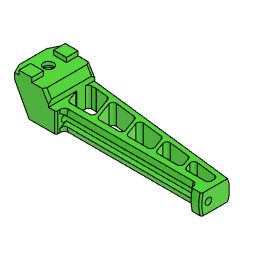
Single Piece Spool Holder v23 (Autodesk Fusion 360 design; units mm, degrees)
Autodesk Fusion 360 part; units mm, degrees
sketch "Sketch1" plane through (0, 0, 0) normal (0, 1, 0) x (1, 0, 0)
  line L0 (0, 0) -> (123.25, 0)
  line L1 (123.25, 0) -> (123.25, -30)
  line L2 (123.25, -30) -> (0, -30)
  line L3 (0, -30) -> (0, 0)
  line L4 (10, -30) -> (10, 0) construction
  line L5 (25, -30) -> (25, 0) construction
  dimension "d2" = 30
  dimension "d39" = 10
  dimension "d40" = 15
  dimension "d74" = 123.25
  constraint horizontal L0
  constraint vertical L1
  constraint horizontal L2
  constraint vertical L3
  constraint coincident L0.start L3.end
  constraint coincident L2 L4.start
  constraint coincident L0 L4.end
  constraint perpendicular L0 L4
  constraint coincident L2 L5.start
  constraint coincident L0 L5.end
  constraint perpendicular L0 L5
  measures "d2" distance of L0.start L2.end
  measures "d39" distance of L3 L4
  measures "d40" distance of L4 L5
  measures "d74" distance of L1 L3
extrude "Extrude1" add sketch "Sketch1" along normal mid plane 13 makes body 1
sketch "Sketch7" plane through (0, 6.5, 0) normal (0, 1, 0) x (-1, 0, 0)
  line L0 (0, 30) -> (-123.25, 30)
  line L1 (-123.25, 30) -> (-123.25, 0)
  line L2 (-123.25, 0) -> (0, 0)
  line L3 (0, 0) -> (0, 30)
  line L4 (0, 30) -> (-25, 30)
  line L5 (-25, 30) -> (-25, 0)
  line L6 (-25, 0) -> (0, 0)
  line L7 (0, 0) -> (0, 30)
  dimension "d75" = 25
  constraint horizontal L4
  constraint vertical L5
  constraint horizontal L6
  constraint vertical L7
  constraint coincident L2 L5.end
  constraint coincident L0.start L3.end
  measures "d75" distance of L0.start L4.end
extrude "Extrude9" add sketch "Sketch7" along normal blind 8.5 contours L0 L2 L3 L4 L5 L6 L7 bodies 1
sketch "Sketch2" plane through (0, 0, 0) normal (0, 0, 1) x (1, 0, 0)
  line L0 (0, -6.5) -> (0, 15)
  line L1 (25, 6.5) -> (123.25, 6.5)
  line L2 (123.25, 6.5) -> (123.25, -6.5)
  line L3 (123.25, -6.5) -> (0, -6.5)
  line L4 (5.825, 15) -> (14.175, 15)
  line L5 (14.175, 15) -> (14.175, 17.8)
  line L6 (14.175, 17.8) -> (5.825, 17.8)
  line L7 (5.825, 17.8) -> (5.825, 15)
  line L8 (10, 17.8) -> (10, 15) construction
  line L9 (0, 15) -> (25, 15)
  line L10 (25, 15) -> (25, 6.5)
  dimension "d20" = 10
  dimension "d21" = 2.8
  dimension "d22" = 8.35
  constraint horizontal L4
  constraint vertical L5
  constraint horizontal L6
  constraint vertical L7
  constraint midpoint L6 L8.start
  constraint midpoint L4 L8.end
  constraint coincident L9 L4.start
  constraint coincident L4.start L7.end
  measures "d20" distance of L0.end L8
  measures "d21" distance of L4.end L5.end
  measures "d22" distance of L5.end L6.end
extrude "Extrude2" add sketch "Sketch2" along normal blind 30 contours L4 L5 L6 L7 L9 bodies 1
sketch "Sketch3" plane through (0, -6.5, 0) normal (0, -1, 0) x (-1, 0, 0)
  line L0 (-10, -30) -> (-10, 0) construction
  circle A0 centre (-10, -15) radius 3.25
  line L1 (-123.25, -30) -> (0, -30)
  line L2 (0, -30) -> (0, 0)
  line L3 (0, 0) -> (-123.25, 0)
  line L4 (-123.25, 0) -> (-123.25, -30)
  line L5 (-14.175, 0) -> (-5.825, 0)
  line L6 (-5.825, 0) -> (-5.825, -30)
  line L7 (-5.825, -30) -> (-14.175, -30)
  line L8 (-14.175, -30) -> (-14.175, 0)
  dimension "d14" = 6.5
  constraint midpoint L0 A0.centre
  constraint midpoint L0.start L7
  constraint midpoint L0.end L5
  measures "d14" diameter of A0
extrude "Extrude3" cut sketch "Sketch3" against normal through all contours A0 bodies 1
sketch "Sketch4" plane through (0, -6.5, 0) normal (0, -1, 0) x (-1, 0, 0)
  circle A0 centre (-10, -15) radius 6.5
  circle A1 centre (-10, -15) radius 3.25
  line L0 (-123.25, -30) -> (0, -30)
  line L1 (0, -30) -> (0, 0)
  line L2 (0, 0) -> (-123.25, 0)
  line L3 (-123.25, 0) -> (-123.25, -30)
  dimension "d16" = 13
  constraint coincident A0.centre A1.centre
  measures "d16" diameter of A0
extrude "Extrude4" cut sketch "Sketch4" against normal up to surface (16 mm away) contours A0 | A1 bodies 1
chamfer "Chamfer1" distance 3.25 angle 45 1 edges at (13.0301, 9.5, 16.1753) on bodies 1
ref_plane "WorkPlane1" through (61.625, 5.65, 15) normal (0, 0, 1) x (1, 0, 0)
sketch "Sketch5" plane through (123.25, 0, 0) normal (1, 0, 0) x (0, 1, 0)
  line L0 (-6.5, 0) -> (6.5, 0)
  line L1 (6.5, 0) -> (6.5, 30)
  line L2 (6.5, 30) -> (-6.5, 30)
  line L3 (-6.5, 30) -> (-6.5, 0)
  circle A0 centre (0, 5.7) radius 20
  circle A1 centre (0, 5.7) radius 24
  line L4 (0, 0) -> (0, 30) construction
  circle A2 centre (0, 24.4) radius 2.1
  line L5 (-6.5, 0) -> (6.5, 0)
  line L6 (6.5, 0) -> (6.5, 30)
  line L7 (6.5, 30) -> (-6.5, 30)
  line L8 (-6.5, 30) -> (-6.5, 0)
  point P0 (27.1204, 5.059)
  point P1 (24.0412, 4.3321)
  point P2 (14.8796, 5.059)
  point P3 (17.9588, 4.3321)
  dimension "d86" = 40
  dimension "d87" = 48
  dimension "d88" = 5.7
  dimension "d89" = 24.4
  dimension "d90" = 4.2
  constraint coincident L4.start origin
  constraint midpoint L2 L4.end
  constraint coincident A0.centre A1.centre
  constraint coincident A0.centre L4
  constraint coincident L4 A2.centre
  measures "d86" diameter of A0
  measures "d87" diameter of A1
  measures "d88" distance of L0 A0.centre
  measures "d89" distance of L4.start A2.centre
  measures "d90" diameter of A2
extrude "Extrude5" cut sketch "Sketch5" against normal blind 86.25 from surface at -7 contours L1 L3 A0 A1 A2 L6 L8 | L1 L2 L3 A1 L6 L7 L8 | A0 A2 picked at (-0.0509, 25.9594) bodies 1
extrude "Extrude6" cut sketch "Sketch5" against normal blind 7 contours L1 L2 L3 A1 L6 L7 L8 bodies 1
extrude "Extrude7" cut sketch "Sketch5" against normal up to surface (100.25 mm away) contours A0 A2 | A0 A2 bodies 1
chamfer "Chamfer2" distance 1.3 distance2 2.2 2 edges at (73.125, -1.7041, 25.6273) (73.125, 1.7041, 25.6273) measured on face at (58.75, -5.4581, 24.9408) measured on face at (58.75, 2.2474, 25.5733) on bodies 1
fillet "Fillet1" radius 1 3 edges at (123.25, 0, 29.7) (116.25, 0, 29.7) (30, 0, 30) on bodies 1
chamfer "Chamfer3" distance 3 distance2 6 2 edges at (0, 4.25, 30) (0, 4.25, 0) measured on face at (18, -2.1667, 30) measured on face at (49.4167, -2.1667, 0) on bodies 1
chamfer "Chamfer4" distance 11 distance2 93 1 edges at (123.25, 0, 0) measured on face at (123.25, 0.0523, 7.4353) on bodies 1
sketch "Sketch6" plane through (0, -6.5, 0) normal (0, -1, 0) x (1, 0, 0)
  line L0 (30, 24.6143) -> (30, 29)
  line L1 (29, 30) -> (3, 30)
  line L2 (3, 30) -> (0, 24)
  line L3 (0, 24) -> (0, 6)
  line L4 (0, 6) -> (3, 0)
  line L5 (3, 0) -> (30.25, 0)
  circle A0 centre (10, 15) radius 6.5
  line L6 (31.5445, 30) -> (20.6254, 0)
  line L7 (29.4161, 30) -> (18.497, 0)
  line L8 (0, 0) -> (128.5239, 0)
  line L9 (128.5239, 0) -> (128.5239, 30)
  line L10 (128.5239, 30) -> (0, 30)
  line L11 (0, 30) -> (0, 0)
  line L12 (48.4161, 30) -> (37.497, 0)
  line L13 (50.5445, 30) -> (39.6254, 0)
  line L14 (67.4161, 30) -> (56.497, 0)
  line L15 (69.5445, 30) -> (58.6254, 0)
  line L16 (86.4161, 30) -> (75.497, 0)
  line L17 (88.5445, 30) -> (77.6254, 0)
  line L18 (105.4161, 30) -> (94.497, 0)
  line L19 (107.5445, 30) -> (96.6254, 0)
  arc A1 (30, 29) -> (29, 30) centre (29, 29) ccw
  line L20 (30.25, 0) -> (123.25, 11)
  line L21 (123.25, 11) -> (123.25, 27.7624)
  spline S0 degree 3 poles (122.25, 28.803) (122.3719, 28.803) (122.5152, 28.7737) (122.7418, 28.6777) (122.8647, 28.5932) (123.0406, 28.4132) (123.1238, 28.285) (123.2204, 28.0461) (123.25, 27.8927) (123.25, 27.7624) knots 0.605058 0.605058 0.605058 0.605058 0.64162 0.64162 0.678904 0.678904 0.71712 0.71712 0.756197 0.756197 0.756197 0.756197
  line L22 (122.25, 28.803) -> (117.25, 28.803)
  spline S1 degree 3 poles (116.25, 27.7624) (116.25, 27.8927) (116.2796, 28.0461) (116.3762, 28.285) (116.4594, 28.4132) (116.6353, 28.5932) (116.7582, 28.6777) (116.9848, 28.7737) (117.1281, 28.803) (117.25, 28.803) knots 0.453919 0.453919 0.453919 0.453919 0.492996 0.492996 0.531212 0.531212 0.568496 0.568496 0.605058 0.605058 0.605058 0.605058
  line L23 (116.25, 27.7624) -> (116.25, 24.6143)
  line L24 (116.25, 24.6143) -> (30, 24.6143)
  line L25 (119.25, 14.5548) -> (119.25, 20.6143)
  line L26 (119.25, 20.6143) -> (26, 20.6143)
  line L27 (26, 20.6143) -> (26, 26)
  line L28 (26, 26) -> (5.4721, 26)
  line L29 (5.4721, 26) -> (4, 23.0557)
  line L30 (4, 23.0557) -> (4, 6.9443)
  line L31 (4, 6.9443) -> (5.4721, 4)
  line L32 (5.4721, 4) -> (30.0143, 4)
  line L33 (30.0143, 4) -> (119.25, 14.5548)
  line L34 (25, 30) -> (25, 0)
  line L35 (116.25, 22.6143) -> (28, 22.6143)
  line L36 (28, 22.6143) -> (28, 29)
  dimension "d51" = 2
  dimension "d55" = 76
  dimension "d56" = 0
  dimension "d59" = 30
  dimension "d61" = 70
  dimension "d101" = -4
  dimension "d108" = -2
  constraint parallel L6 L7
  constraint horizontal L8
  constraint vertical L9
  constraint horizontal L10
  constraint vertical L11
  constraint coincident L8.start L11.end
  constraint coincident L7.start L10
  constraint coincident L6.start L10
  constraint coincident L7.end L8
  constraint coincident L6.end L8
  constraint coincident L7 L26.end
  measures "d51" distance of L6 L7
  measures "d59" distance of L8 L10
  measures "d61" angle of L7 L10
extrude "Extrude8" cut sketch "Sketch6" against normal blind 47 contours L6 L12 L26 L32 L33 L34 | L13 L14 L26 L33 | L15 L16 L26 L33 | L17 L18 L26 L33 | L19 L25 L26 L33 bodies 1
fillet "Fillet2" radius 2 22 edges at (28.1284, 0, 20.6143) (39.355, 0, 5.1048) (61.4339, 0, 7.7163) (79.0645, 0, 9.8016) (101.1434, 0, 12.4131) (119.25, 0, 14.5548) (119.25, 0, 20.6143) (104.1284, 0, 20.6143) (102, 0, 20.6143) (85.1284, 0, 20.6143) (83, 0, 20.6143) (66.1284, 0, 20.6143) (64, 0, 20.6143) (47.1284, 0, 20.6143) (45, 0, 20.6143) (30.0143, 0, 4) (25, 0, 12.0192) (25, 0, 4) (41.5791, 0, 5.3679) (81.2886, 0, 10.0647) (98.9193, 0, 12.1501) (59.2098, 0, 7.4532) on bodies 1
chamfer "Chamfer5" distance 3 distance2 1 2 edges at (76.75, -6.5, 5.5) (76.75, 6.5, 5.5) measured on face at (61.25, 2.1667, 3.6667) measured on face at (61.25, 2.1667, 3.6667) on bodies 1
chamfer "Chamfer6" distance 2 distance2 5 1 edges at (12.3683, -6.5, 0) measured on face at (14.7916, -6.5, 27.0169) on bodies 1
chamfer "Chamfer7" distance 9 distance2 17 1 edges at (0, -6.5, 15) measured on face at (14.7916, -6.5, 27.0169) on bodies 1
fillet "Fillet3" radius 2.5 4 edges at (30, -4.767, 25.1236) (30, 4.767, 25.1236) (116.25, -4.767, 25.1236) (116.25, 4.767, 25.1236) on bodies 1
chamfer "Chamfer12" distance 3 distance2 3 2 edges at (6, -0.8333, 30) (7.6765, -4, 1) measured on face at (6.2596, -1.3237, 26.8819) measured on face at (6.2596, -1.3237, 26.8819) on bodies 1
sketch "Sketch8" plane through (0, 17.8, 0) normal (0, 1, 0) x (-1, 0, 0)
  circle A0 centre (-10, 15) radius 3.25
  line L0 (-14.175, 0) -> (-5.825, 0)
  line L1 (-5.825, 0) -> (-5.825, 30)
  line L2 (-5.825, 30) -> (-14.175, 30)
  line L3 (-14.175, 30) -> (-14.175, 0)
  line L4 (-5.825, 22.5) -> (-14.175, 22.5)
  line L5 (-14.175, 22.5) -> (-14.175, 7.5)
  line L6 (-14.175, 7.5) -> (-5.825, 7.5)
  line L7 (-5.825, 7.5) -> (-5.825, 22.5)
  line L8 (-5.825, 22.5) -> (-14.175, 7.5) construction
  line L9 (-14.175, 22.5) -> (-5.825, 7.5) construction
  point P0 (-10, 15)
  dimension "d93" = 15
  constraint horizontal L4
  constraint perpendicular L4 L5
  constraint parallel L4 L6
  constraint parallel L5 L7
  constraint coincident L1 L4.start
  constraint coincident L8 P0
  constraint coincident L9 P0
  constraint coincident P0 A0.centre
  measures "d93" distance of L4.start L6.end
extrude "Extrude10" cut sketch "Sketch8" against normal up to surface (2.8 mm away) contours L1 L3 L4 L5 L6 L7 bodies 1
sketch "Sketch9" plane through (123.25, 0, 0) normal (1, 0, 0) x (0, 1, 0)
  arc A0 (6.5, 27.7624) -> (-6.5, 27.7624) centre (0, 5.7) ccw
  circle A1 centre (0, 24.4) radius 2
  circle A2 centre (0, 24.4) radius 1
  line L0 (3.5, 11) -> (6.5, 12.007)
  line L1 (6.5, 12.007) -> (6.5, 27.7624)
  line L2 (-6.5, 27.7624) -> (-6.5, 12.007)
  line L3 (-6.5, 12.007) -> (-3.5, 11)
  line L4 (-3.5, 11) -> (3.5, 11)
  circle A3 centre (0, 24.4) radius 2.1
  dimension "d96" = 4
  dimension "d97" = 2
  measures "d96" diameter of A1
  measures "d97" diameter of A2
extrude "Extrude11" add sketch "Sketch9" against normal blind 100.25 separate body contours A1 makes body 2
chamfer "Chamfer13" distance 3 distance2 5 1 edges at (25, 15, 15) measured on face at (21.0833, 15, 15) on bodies 1
chamfer "Chamfer14" distance 2 distance2 1 2 edges at (23.5, 12.5, 30) (23.5, 12.5, 0) measured on face at (23, 13.3333, 20) measured on face at (23, 13.3333, 20) on bodies 1
move_body "Move1" bodies 1 to x (1, 0, 0) y (0, 0, 1) z (0, -1, 0) at (0, 23.5, 36.5)
hidden bodies 2
named bodies: "Single Piece Spool Holder"
